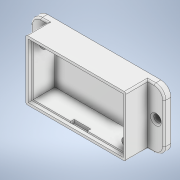
# Autodesk Inventor part: case_down
Saved by Autodesk Inventor 2022 (Build 260153000, 153)
## iProperties
Created: 2022-01-07
Part Number: case_down
Material: Пластик АБС
Document SubType Name: Modeling
Designer: Me
Density: 1.06 g/cm^3
Appearance: Гладкий — белый
Author: Me
Autodesk Inventor part; units mm, degrees
ref_plane "YZ Plane" through (0, 0, 0) normal (1, 0, 0) x (0, 1, 0)
ref_plane "XZ Plane" through (0, 0, 0) normal (0, 1, 0) x (-1, 0, 0)
ref_plane "XY Plane" through (0, 0, 0) normal (0, 0, 1) x (1, 0, 0)
sketch "Эскиз1" plane through (0, 0, 0) normal (0, 0, 1) x (1, 0, 0)
  line L0 (-34, 18) -> (34, 18)
  line L1 (40, 12) -> (40, -12)
  line L2 (34, -18) -> (-34, -18)
  line L3 (-40, -12) -> (-40, 12)
  line L4 (-783.3238, 613.5811) -> (-63.593, 613.5811) construction
  line L5 (-63.593, 613.5811) -> (-63.593, 43.008) construction
  line L6 (-63.593, 43.008) -> (-783.3238, 43.008) construction
  line L7 (-783.3238, 43.008) -> (-783.3238, 613.5811) construction
  arc A0 (-34, 18) -> (-40, 12) centre (-34, 12) ccw
  arc A1 (-40, -12) -> (-34, -18) centre (-34, -12) ccw
  arc A2 (40, 12) -> (34, 18) centre (34, 12) ccw
  arc A3 (34, -18) -> (40, -12) centre (34, -12) ccw
  point P0 (0, 0)
  point P1 (-40, 18)
  point P2 (40, 18)
  point P3 (-40, -18)
  dimension "d1" = 80
  dimension "d4" = 40
  dimension "d5" = 36
  dimension "d6" = 18
  dimension "d7" = 6
  dimension "d8" = 6
  dimension "d9" = 6
  constraints: 8 end point, 8 point on circle, 8 tangent, 6 point on line, 4 centre point, 2 parallel, 1 equal radius, 1 horizontal, 1 perpendicular, 2 other
  measures "d1" distance of point (-40, 18) point (40, 18)
  measures "d4" distance from line of point (0, 0) L3
  measures "d5" distance of point (-40, -18) point (-40, 18)
  measures "d6" distance from line of point (0, 0) L0
  measures "d7" radius of A0
  measures "d8" radius of A1
  measures "d9" radius of A2
extrude "Выдавливание1" add sketch "Эскиз1" along normal blind 4
sketch "Эскиз2" plane through (0, 0, 4) normal (0, 0, 1) x (1, 0, 0)
  line L0 (-29, 18) -> (29, 18)
  line L1 (30, 17) -> (30, -17)
  line L2 (29, -18) -> (-29, -18)
  line L3 (-30, -17) -> (-30, 17)
  line L4 (-40, 12) -> (-40, -12) projected
  line L5 (40, -12) -> (40, 12) projected
  line L6 (34, 18) -> (-34, 18) projected
  line L7 (-34, -18) -> (34, -18) projected
  arc A0 (-29, 18) -> (-30, 17) centre (-29, 17) ccw
  arc A1 (-30, -17) -> (-29, -18) centre (-29, -17) ccw
  arc A2 (29, -18) -> (30, -17) centre (29, -17) ccw
  arc A3 (30, 17) -> (29, 18) centre (29, 17) ccw
  point P0 (0, 0)
  dimension "d12" = 10
  dimension "d13" = 10
  dimension "d14" = 0
  dimension "d15" = 0
  dimension "d16" = 1
  constraints: 8 end point, 8 point on circle, 8 tangent, 4 centre point, 3 equal radius, 2 parallel, 1 horizontal, 1 perpendicular
  measures "d12" distance between parallel lines of L4 L3
  measures "d13" distance between parallel lines of L5 L1
  measures "d14" distance between parallel lines of L6 L0
  measures "d15" distance between parallel lines of L7 L2
  measures "d16" radius of A0
extrude "Выдавливание2" add sketch "Эскиз2" along normal blind 13
sketch "Эскиз3" plane through (0, 0, 17) normal (0, 0, 1) x (1, 0, 0)
  line L0 (-27.5, 15.5) -> (27.5, 15.5)
  line L1 (27.5, 15.5) -> (27.5, -15.5)
  line L2 (27.5, -15.5) -> (-27.5, -15.5)
  line L3 (-27.5, -15.5) -> (-27.5, 15.5)
  line L4 (29, 18) -> (-29, 18) projected
  line L5 (-29, -18) -> (29, -18) projected
  line L6 (30, -17) -> (30, 17) projected
  line L7 (-30, 17) -> (-30, -17) projected
  point P0 (0, 0)
  dimension "d19" = 2.5
  dimension "d20" = 2.5
  dimension "d21" = 2.5
  dimension "d22" = 2.5
  constraints: 8 end point, 2 parallel, 1 horizontal, 1 perpendicular
  measures "d19" distance between parallel lines of L4 L0
  measures "d20" distance between parallel lines of L5 L2
  measures "d21" distance between parallel lines of L6 L1
  measures "d22" distance between parallel lines of L7 L3
extrude "Выдавливание3" cut sketch "Эскиз3" against normal blind 15
sketch "Эскиз4" plane through (0, 0, 4) normal (0, 0, 1) x (1, 0, 0)
  circle A0 centre (-35, 0) radius 2.25
  circle A1 centre (35, 0) radius 2.25
  line L0 (-40, 12) -> (-40, -12) projected
  line L1 (40, -12) -> (40, 12) projected
  point P0 (0, 0)
  dimension "d25" = 4.5
  dimension "d26" = 4.5
  dimension "d27" = 5
  dimension "d28" = 5
  constraints: 2 centre point
  measures "d25" diameter of A0
  measures "d26" diameter of A1
  measures "d27" distance from line of L0 A0.centre
  measures "d28" distance from line of L1 A1.centre
extrude "Выдавливание4" cut sketch "Эскиз4" against normal through all
chamfer "Фаска1" distance 1 angle 45 2 edges at (-37.25, 0, 4) (32.75, 0, 4)
sketch "Эскиз5" plane through (0, 0, 17) normal (0, 0, 1) x (1, 0, 0)
  line L0 (-28.5, 16.5) -> (28.5, 16.5)
  line L1 (28.5, 16.5) -> (28.5, -16.5)
  line L2 (28.5, -16.5) -> (-28.5, -16.5)
  line L3 (-28.5, -16.5) -> (-28.5, 16.5)
  line L4 (29, 18) -> (-29, 18) projected
  line L5 (30, -17) -> (30, 17) projected
  line L6 (-29, -18) -> (29, -18) projected
  line L7 (-30, 17) -> (-30, -17) projected
  point P0 (0, 0)
  dimension "d34" = 1.5
  dimension "d35" = 1.5
  dimension "d36" = 1.5
  dimension "d37" = 1.5
  constraints: 8 end point, 2 parallel, 1 horizontal, 1 perpendicular
  measures "d34" distance between parallel lines of L4 L0
  measures "d35" distance between parallel lines of L5 L1
  measures "d36" distance between parallel lines of L6 L2
  measures "d37" distance between parallel lines of L7 L3
extrude "Выдавливание5" cut sketch "Эскиз5" against normal blind 2 draft -3
sketch "Эскиз6" plane through (-27.5, 15.5, 2) normal (0, -1, 0) x (1, 0, 0)
  line L0 (22.5, 13) -> (32.5, 13)
  line L1 (32.5, 13) -> (32.5, 11)
  line L2 (32.5, 11) -> (22.5, 11)
  line L3 (22.5, 11) -> (22.5, 13)
  line L4 (55, 13) -> (0, 13) projected
  line L5 (55, 13) -> (55, 0) projected
  point P0 (27.5, -2)
  dimension "d40" = 10
  dimension "d41" = 0
  dimension "d42" = 2
  dimension "d45" = 22.5
  constraints: 8 end point, 2 parallel, 1 horizontal, 1 perpendicular
  measures "d40" distance of L0.start L0.end
  measures "d41" distance between parallel lines of L4 L0
  measures "d42" distance of L0.end L1.end
  measures "d45" distance between parallel lines of L5 L1
extrude "Выдавливание6" cut sketch "Эскиз6" against normal blind 2
sketch "Эскиз7" plane through (-27.5, -15.5, 2) normal (0, 1, 0) x (1, 0, 0)
  line L0 (32.5, -13) -> (22.5, -13)
  line L1 (22.5, -13) -> (22.5, -11)
  line L2 (22.5, -11) -> (32.5, -11)
  line L3 (32.5, -11) -> (32.5, -13)
  line L4 (0, -13) -> (55, -13) projected
  line L5 (0, -13) -> (0, 0) projected
  point P0 (27.5, 2)
  dimension "d46" = 10
  dimension "d47" = 2
  dimension "d48" = 0
  dimension "d49" = 22.5
  constraints: 8 end point, 2 parallel, 1 horizontal, 1 perpendicular
  measures "d46" distance of L0.start L0.end
  measures "d47" distance of L0.end L1.end
  measures "d48" distance between parallel lines of L4 L0
  measures "d49" distance between parallel lines of L5 L1
extrude "Выдавливание7" cut sketch "Эскиз7" against normal blind 2
fillet "Сопряжение1" radius 1 10 edges at (-38.2426, -16.2426, 4) (-31.5, -18, 4) (-38.2426, 16.2426, 4) (-31.5, 18, 4) (-40, 0, 4) (38.2426, 16.2426, 4) (31.5, 18, 4) (38.2426, -16.2426, 4) (31.5, -18, 4) (40, 0, 4)
sketch "Эскиз10" plane through (0, 0, 2) normal (0, 0, 1) x (1, 0, 0)
  circle A0 centre (-25, 13) radius 2.5
  line L0 (-27.5, -15.5) -> (-27.5, 15.5) projected
  line L1 (-27.5, 15.5) -> (27.5, 15.5) projected
  circle A1 centre (25, -13) radius 2.5
  line L2 (27.5, 15.5) -> (27.5, -15.5) projected
  line L3 (27.5, -15.5) -> (-27.5, -15.5) projected
  point P0 (0, 0)
  dimension "d69" = 5
  dimension "d70" = 2.5
  dimension "d71" = 2.5
  dimension "d72" = 2.5
  dimension "d73" = 2.5
  dimension "d74" = 5
  constraints: 2 centre point
  measures "d69" diameter of A0
  measures "d70" distance from line of L0 A0.centre
  measures "d71" distance from line of L1 A0.centre
  measures "d72" distance from line of L2 A1.centre
  measures "d73" distance from line of L3 A1.centre
  measures "d74" diameter of A1
extrude "Выдавливание10" add sketch "Эскиз10" along normal blind 10 contours A0 | A1
sketch "Эскиз11" plane through (0, 0, 12) normal (0, 0, 1) x (1, 0, 0)
  circle A0 centre (-25, 13) radius 1
  circle A1 centre (25, -13) radius 1
  arc A2 (-27.5, 13) -> (-25, 15.5) centre (-25, 13) ccw projected
  arc A3 (27.5, -13) -> (25, -15.5) centre (25, -13) ccw projected
  point P0 (0, 0)
  dimension "d77" = 0
  dimension "d78" = 0
  dimension "d79" = 2
  dimension "d80" = 0
  dimension "d81" = 0
  dimension "d82" = 2
  constraints: 2 centre point
  measures "d77" distance of A2.centre A0.centre
  measures "d78" distance of A2.centre A0.centre
  measures "d79" diameter of A0
  measures "d80" distance of A3.centre A1.centre
  measures "d81" distance of A3.centre A1.centre
  measures "d82" diameter of A1
extrude "Выдавливание11" cut sketch "Эскиз11" against normal blind 10
thread "Резьба1" size "M2x0.4" class "6H" standard "ANSI Metric M Profile" full length
thread "Резьба2" size "M2x0.4" class "6H" standard "ANSI Metric M Profile" full length
